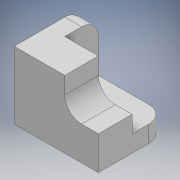
# Autodesk Inventor part: 36
Saved by Autodesk Inventor 2017 (Build 210142000, 142)
## iProperties
Part Number: 36
Material: 一般
Document SubType Name: Modeling
Designer: Brian
Density: 1 g/cm^3
Appearance: 預設
Author: Brian
Autodesk Inventor part; units mm, degrees
ref_plane "YZ Plane" through (0, 0, 0) normal (1, 0, 0) x (0, 1, 0)
ref_plane "XZ Plane" through (0, 0, 0) normal (0, 1, 0) x (-1, 0, 0)
ref_plane "XY Plane" through (0, 0, 0) normal (0, 0, 1) x (1, 0, 0)
sketch "草圖1" plane through (0, 0, 0) normal (0, 1, 0) x (-1, 0, 0)
  line L0 (0, 0) -> (-30, 0)
  line L1 (-30, 0) -> (-30, -40)
  line L2 (-30, -40) -> (0, -40)
  line L3 (0, -40) -> (0, 0)
  line L4 (-30, -40) -> (-50, -40)
  line L5 (-50, -40) -> (-50, -20)
  line L6 (-50, -20) -> (-30, -20)
  line L7 (-30, -20) -> (-30, -40)
  dimension "d0" = 40
  dimension "d1" = 20
  dimension "d2" = 20
  dimension "d3" = 30
  constraints: 16 end point, 4 parallel, 2 horizontal, 2 perpendicular
  measures "d0" distance of L2.end L0.start
  measures "d1" distance of L4.end L5.end
  measures "d2" distance of L5.end L6.end
  measures "d3" distance of L1.end L2.end
extrude "擠出1" add sketch "草圖1" along normal blind 20
sketch "草圖2" plane through (0, 0, -40) normal (-1, 0, 0) x (0, 0, 1)
  line L0 (40, 0) -> (40, 20) projected
  line L1 (40, 20) -> (0, 20)
  line L2 (0, 20) -> (0, 40)
  line L3 (0, 40) -> (40, 40)
  line L4 (40, 40) -> (40, 20)
  dimension "d6" = 20
  constraints: 8 end point, 2 parallel, 1 horizontal, 1 perpendicular
  measures "d6" distance of L1.end L2.end
extrude "擠出2" add sketch "草圖2" against normal blind 10
sketch "草圖3" plane through (50, 0, -40) normal (0, 0, -1) x (-1, 0, 0)
  line L0 (0, 20) -> (40, 20) projected
  line L1 (50, 40) -> (40, 40) projected
  line L2 (0, 20) -> (40, 20)
  line L3 (40, 20) -> (40, 40)
  line L4 (40, 40) -> (0, 40)
  line L5 (0, 40) -> (0, 20)
  point P0 (50, 0)
  constraints: 8 end point, 2 parallel, 1 horizontal, 1 perpendicular
extrude "擠出3" add sketch "草圖3" against normal blind 10
fillet "圓角1" radius 10 3 edges at (50, 40, -35) (5, 40, 0) (30, 10, -20)
